Autodesk Fusion 360 part; units mm, degrees
(part 5 of 7)
  spline S7 degree 5 poles (-6.1927, -9.0912) (-6.1879, -9.089) (-6.1784, -9.0847) (-6.164, -9.0781) (-6.1449, -9.0692) (-6.1211, -9.0581) (-6.0974, -9.0469) (-6.0739, -9.0356) (-6.0504, -9.0242) (-6.0269, -9.0127) (-6.0036, -9.0011) (-5.9804, -8.9894) (-5.9573, -8.9776) (-5.9343, -8.9657) (-5.9113, -8.9538) (-5.8885, -8.9417) (-5.8657, -8.9295) (-5.8431, -8.9173) (-5.8206, -8.9049) (-5.7981, -8.8925) (-5.7758, -8.8799) (-5.7536, -8.8673) (-5.7314, -8.8545) (-5.7094, -8.8417) (-5.6875, -8.8288) (-5.6657, -8.8158) (-5.644, -8.8026) (-5.6224, -8.7894) (-5.6009, -8.7761) (-5.5795, -8.7627) (-5.5583, -8.7492) (-5.5371, -8.7356) (-5.5161, -8.7218) (-5.4952, -8.708) (-5.4744, -8.6941) (-5.4537, -8.6801) (-5.4331, -8.666) (-5.4127, -8.6518) (-5.3924, -8.6375) (-5.3722, -8.6231) (-5.3522, -8.6085) (-5.3323, -8.5939) (-5.3125, -8.5792) (-5.2928, -8.5643) (-5.2733, -8.5494) (-5.2539, -8.5343) (-5.2347, -8.5192) (-5.2156, -8.5039) (-5.1966, -8.4885) (-5.1778, -8.473) (-5.1592, -8.4574) (-5.1407, -8.4417) (-5.1224, -8.4258) (-5.1042, -8.4099) (-5.0862, -8.3938) (-5.0684, -8.3776) (-5.0507, -8.3612) (-5.0332, -8.3448) (-5.0159, -8.3283) (-4.9987, -8.3116) (-4.9818, -8.2947) (-4.9651, -8.2777) (-4.9487, -8.2605) (-4.9326, -8.2431) (-4.9167, -8.2256) (-4.901, -8.2079) (-4.8854, -8.1901) (-4.87, -8.1723) (-4.8548, -8.1543) (-4.84, -8.1361) (-4.8257, -8.1175) (-4.8149, -8.1023) (-4.8073, -8.0905) (-4.8024, -8.0825) (-4.8, -8.0785) knots -1 -1 -1 -1 -1 -1 -0.98571429 -0.97142857 -0.95714286 -0.94285714 -0.92857143 -0.91428571 -0.9 -0.88571429 -0.87142857 -0.85714286 -0.84285714 -0.82857143 -0.81428571 -0.8 -0.78571429 -0.77142857 -0.75714286 -0.74285714 -0.72857143 -0.71428571 -0.7 -0.68571429 -0.67142857 -0.65714286 -0.64285714 -0.62857143 -0.61428571 -0.6 -0.58571429 -0.57142857 -0.55714286 -0.54285714 -0.52857143 -0.51428571 -0.5 -0.48571429 -0.47142857 -0.45714286 -0.44285714 -0.42857143 -0.41428571 -0.4 -0.38571429 -0.37142857 -0.35714286 -0.34285714 -0.32857143 -0.31428571 -0.3 -0.28571429 -0.27142857 -0.25714286 -0.24285714 -0.22857143 -0.21428571 -0.2 -0.18571429 -0.17142857 -0.15714286 -0.14285714 -0.12857143 -0.11428571 -0.1 -0.08571429 -0.07142857 -0.05714286 -0.04285714 -0.02857143 -0.01428571 0 0 0 0 0 0
  line L7 (-4.8, -8.0785) -> (-4.6678, -7.856)
  arc A15 (-4.2652, -7.7464) -> (-4.6678, -7.856) centre (-4.4099, -8.0092) ccw
  arc A16 (-4.2652, -7.7464) -> (-3.76, -8.0038) centre (0, 0) ccw
  arc A17 (-3.6119, -8.3939) -> (-3.76, -8.0038) centre (-3.8875, -8.2754) ccw
  line L8 (-3.6119, -8.3939) -> (-3.7143, -8.6317)
  spline S8 degree 5 poles (-3.7143, -8.6317) (-3.7161, -8.636) (-3.7197, -8.6447) (-3.7247, -8.6577) (-3.7308, -8.6754) (-3.7374, -8.6979) (-3.7434, -8.7206) (-3.749, -8.7435) (-3.7544, -8.7664) (-3.7596, -8.7895) (-3.7647, -8.8126) (-3.7695, -8.8357) (-3.7741, -8.859) (-3.7784, -8.8824) (-3.7824, -8.9059) (-3.786, -8.9295) (-3.7894, -8.9532) (-3.7926, -8.9769) (-3.7956, -9.0007) (-3.7984, -9.0246) (-3.8011, -9.0486) (-3.8035, -9.0726) (-3.8058, -9.0967) (-3.8079, -9.1208) (-3.8097, -9.145) (-3.8114, -9.1693) (-3.8128, -9.1936) (-3.8141, -9.218) (-3.8153, -9.2424) (-3.8162, -9.2669) (-3.817, -9.2914) (-3.8176, -9.316) (-3.8181, -9.3406) (-3.8184, -9.3653) (-3.8185, -9.39) (-3.8185, -9.4147) (-3.8183, -9.4395) (-3.8179, -9.4644) (-3.8174, -9.4893) (-3.8168, -9.5142) (-3.8159, -9.5391) (-3.815, -9.5641) (-3.8139, -9.5892) (-3.8126, -9.6142) (-3.8112, -9.6394) (-3.8096, -9.6645) (-3.8079, -9.6897) (-3.806, -9.7149) (-3.804, -9.7401) (-3.8019, -9.7654) (-3.7996, -9.7907) (-3.7972, -9.816) (-3.7946, -9.8414) (-3.7919, -9.8668) (-3.7891, -9.8922) (-3.7861, -9.9176) (-3.783, -9.9431) (-3.7797, -9.9686) (-3.7763, -9.9941) (-3.7728, -10.0197) (-3.7692, -10.0452) (-3.7654, -10.0708) (-3.7614, -10.0964) (-3.7574, -10.1221) (-3.7532, -10.1477) (-3.7489, -10.1734) (-3.7444, -10.1991) (-3.7398, -10.2248) (-3.7351, -10.2506) (-3.7303, -10.2763) (-3.7253, -10.3021) (-3.7212, -10.3227) (-3.7181, -10.3382) (-3.716, -10.3485) (-3.7149, -10.3537) knots 0 0 0 0 0 0 0.01428571 0.02857143 0.04285714 0.05714286 0.07142857 0.08571429 0.1 0.11428571 0.12857143 0.14285714 0.15714286 0.17142857 0.18571429 0.2 0.21428571 0.22857143 0.24285714 0.25714286 0.27142857 0.28571429 0.3 0.31428571 0.32857143 0.34285714 0.35714286 0.37142857 0.38571429 0.4 0.41428571 0.42857143 0.44285714 0.45714286 0.47142857 0.48571429 0.5 0.51428571 0.52857143 0.54285714 0.55714286 0.57142857 0.58571429 0.6 0.61428571 0.62857143 0.64285714 0.65714286 0.67142857 0.68571429 0.7 0.71428571 0.72857143 0.74285714 0.75714286 0.77142857 0.78571429 0.8 0.81428571 0.82857143 0.84285714 0.85714286 0.87142857 0.88571429 0.9 0.91428571 0.92857143 0.94285714 0.95714286 0.97142857 0.98571429 1 1 1 1 1 1
  arc A18 (-3.7149, -10.3537) -> (-3.0803, -10.5599) centre (0, 0) ccw
  spline S9 degree 5 poles (-3.0803, -10.5599) (-3.0764, -10.5564) (-3.0687, -10.5492) (-3.057, -10.5385) (-3.0416, -10.5242) (-3.0224, -10.5063) (-3.0034, -10.4883) (-2.9844, -10.4703) (-2.9656, -10.4522) (-2.9469, -10.434) (-2.9283, -10.4158) (-2.9098, -10.3975) (-2.8915, -10.3791) (-2.8732, -10.3607) (-2.8551, -10.3422) (-2.8371, -10.3237) (-2.8193, -10.3051) (-2.8015, -10.2864) (-2.7839, -10.2677) (-2.7664, -10.249) (-2.7491, -10.2301) (-2.7318, -10.2112) (-2.7147, -10.1923) (-2.6977, -10.1733) (-2.6809, -10.1542) (-2.6642, -10.1351) (-2.6476, -10.1159) (-2.6311, -10.0966) (-2.6148, -10.0773) (-2.5986, -10.058) (-2.5826, -10.0386) (-2.5667, -10.0191) (-2.5509, -9.9995) (-2.5353, -9.9799) (-2.5198, -9.9603) (-2.5045, -9.9406) (-2.4893, -9.9208) (-2.4743, -9.901) (-2.4594, -9.8811) (-2.4446, -9.8611) (-2.43, -9.8411) (-2.4156, -9.821) (-2.4014, -9.8009) (-2.3873, -9.7807) (-2.3733, -9.7605) (-2.3595, -9.7402) (-2.3459, -9.7198) (-2.3325, -9.6994) (-2.3192, -9.6789) (-2.3061, -9.6584) (-2.2932, -9.6378) (-2.2805, -9.6171) (-2.2679, -9.5964) (-2.2556, -9.5755) (-2.2435, -9.5547) (-2.2315, -9.5338) (-2.2198, -9.5128) (-2.2082, -9.4917) (-2.1968, -9.4706) (-2.1856, -9.4495) (-2.1747, -9.4282) (-2.1641, -9.4069) (-2.1539, -9.3855) (-2.1439, -9.3639) (-2.1342, -9.3423) (-2.1248, -9.3207) (-2.1154, -9.299) (-2.1063, -9.2772) (-2.0974, -9.2554) (-2.0889, -9.2335) (-2.0811, -9.2115) (-2.0755, -9.1936) (-2.0719, -9.1801) (-2.0697, -9.171) (-2.0687, -9.1664) knots -1 -1 -1 -1 -1 -1 -0.98571429 -0.97142857 -0.95714286 -0.94285714 -0.92857143 -0.91428571 -0.9 -0.88571429 -0.87142857 -0.85714286 -0.84285714 -0.82857143 -0.81428571 -0.8 -0.78571429 -0.77142857 -0.75714286 -0.74285714 -0.72857143 -0.71428571 -0.7 -0.68571429 -0.67142857 -0.65714286 -0.64285714 -0.62857143 -0.61428571 -0.6 -0.58571429 -0.57142857 -0.55714286 -0.54285714 -0.52857143 -0.51428571 -0.5 -0.48571429 -0.47142857 -0.45714286 -0.44285714 -0.42857143 -0.41428571 -0.4 -0.38571429 -0.37142857 -0.35714286 -0.34285714 -0.32857143 -0.31428571 -0.3 -0.28571429 -0.27142857 -0.25714286 -0.24285714 -0.22857143 -0.21428571 -0.2 -0.18571429 -0.17142857 -0.15714286 -0.14285714 -0.12857143 -0.11428571 -0.1 -0.08571429 -0.07142857 -0.05714286 -0.04285714 -0.02857143 -0.01428571 0 0 0 0 0 0
  line L9 (-2.0687, -9.1664) -> (-2.0117, -8.9139)
  arc A19 (-1.6627, -8.6853) -> (-2.0117, -8.9139) centre (-1.7191, -8.9799) ccw
  arc A20 (-1.6627, -8.6853) -> (-1.1026, -8.774) centre (0, 0) ccw
  arc A21 (-0.8413, -9.0993) -> (-1.1026, -8.774) centre (-1.14, -9.0716) ccw
  line L10 (-0.8413, -9.0993) -> (-0.8651, -9.357)
  spline S10 degree 5 poles (-0.8651, -9.357) (-0.8655, -9.3617) (-0.8663, -9.371) (-0.867, -9.385) (-0.8673, -9.4037) (-0.8667, -9.4271) (-0.8654, -9.4506) (-0.8636, -9.474) (-0.8616, -9.4975) (-0.8595, -9.5211) (-0.8572, -9.5446) (-0.8546, -9.5681) (-0.8518, -9.5917) (-0.8487, -9.6152) (-0.8452, -9.6388) (-0.8414, -9.6624) (-0.8373, -9.686) (-0.833, -9.7095) (-0.8285, -9.7331) (-0.8238, -9.7567) (-0.8189, -9.7803) (-0.8138, -9.8039) (-0.8085, -9.8275) (-0.803, -9.8511) (-0.7973, -9.8747) (-0.7914, -9.8983) (-0.7853, -9.9219) (-0.779, -9.9454) (-0.7725, -9.969) (-0.7658, -9.9926) (-0.759, -10.0162) (-0.752, -10.0397) (-0.7448, -10.0633) (-0.7375, -10.0868) (-0.73, -10.1104) (-0.7223, -10.1339) (-0.7144, -10.1574) (-0.7064, -10.181) (-0.6982, -10.2045) (-0.6899, -10.228) (-0.6814, -10.2515) (-0.6728, -10.2749) (-0.664, -10.2984) (-0.655, -10.3218) (-0.6459, -10.3453) (-0.6367, -10.3687) (-0.6273, -10.3921) (-0.6177, -10.4155) (-0.608, -10.4389) (-0.5982, -10.4623) (-0.5882, -10.4857) (-0.578, -10.509) (-0.5678, -10.5323) (-0.5573, -10.5556) (-0.5468, -10.5789) (-0.5361, -10.6022) (-0.5252, -10.6255) (-0.5143, -10.6487) (-0.5032, -10.6719) (-0.4919, -10.6951) (-0.4805, -10.7183) (-0.469, -10.7415) (-0.4574, -10.7646) (-0.4456, -10.7878) (-0.4337, -10.8109) (-0.4216, -10.834) (-0.4094, -10.857) (-0.3971, -10.8801) (-0.3847, -10.9031) (-0.3721, -10.9261) (-0.3594, -10.9491) (-0.3492, -10.9674) (-0.3414, -10.9812) (-0.3362, -10.9904) (-0.3336, -10.9949) knots 0 0 0 0 0 0 0.01428571 0.02857143 0.04285714 0.05714286 0.07142857 0.08571429 0.1 0.11428571 0.12857143 0.14285714 0.15714286 0.17142857 0.18571429 0.2 0.21428571 0.22857143 0.24285714 0.25714286 0.27142857 0.28571429 0.3 0.31428571 0.32857143 0.34285714 0.35714286 0.37142857 0.38571429 0.4 0.41428571 0.42857143 0.44285714 0.45714286 0.47142857 0.48571429 0.5 0.51428571 0.52857143 0.54285714 0.55714286 0.57142857 0.58571429 0.6 0.61428571 0.62857143 0.64285714 0.65714286 0.67142857 0.68571429 0.7 0.71428571 0.72857143 0.74285714 0.75714286 0.77142857 0.78571429 0.8 0.81428571 0.82857143 0.84285714 0.85714286 0.87142857 0.88571429 0.9 0.91428571 0.92857143 0.94285714 0.95714286 0.97142857 0.98571429 1 1 1 1 1 1
  arc A22 (-0.3336, -10.9949) -> (0.3336, -10.9949) centre (0, 0) ccw
  spline S11 degree 5 poles (0.3336, -10.9949) (0.3362, -10.9904) (0.3414, -10.9812) (0.3492, -10.9674) (0.3594, -10.9491) (0.3721, -10.9261) (0.3847, -10.9031) (0.3971, -10.8801) (0.4094, -10.857) (0.4216, -10.834) (0.4337, -10.8109) (0.4456, -10.7878) (0.4574, -10.7646) (0.469, -10.7415) (0.4805, -10.7183) (0.4919, -10.6951) (0.5032, -10.6719) (0.5143, -10.6487) (0.5252, -10.6255) (0.5361, -10.6022) (0.5468, -10.5789) (0.5573, -10.5556) (0.5678, -10.5323) (0.578, -10.509) (0.5882, -10.4857) (0.5982, -10.4623) (0.608, -10.4389) (0.6177, -10.4155) (0.6273, -10.3921) (0.6367, -10.3687) (0.6459, -10.3453) (0.655, -10.3218) (0.664, -10.2984) (0.6728, -10.2749) (0.6814, -10.2515) (0.6899, -10.228) (0.6982, -10.2045) (0.7064, -10.181) (0.7144, -10.1574) (0.7223, -10.1339) (0.73, -10.1104) (0.7375, -10.0868) (0.7448, -10.0633) (0.752, -10.0397) (0.759, -10.0162) (0.7658, -9.9926) (0.7725, -9.969) (0.779, -9.9454) (0.7853, -9.9219) (0.7914, -9.8983) (0.7973, -9.8747) (0.803, -9.8511) (0.8085, -9.8275) (0.8138, -9.8039) (0.8189, -9.7803) (0.8238, -9.7567) (0.8285, -9.7331) (0.833, -9.7095) (0.8373, -9.686) (0.8414, -9.6624) (0.8452, -9.6388) (0.8487, -9.6152) (0.8518, -9.5917) (0.8546, -9.5681) (0.8572, -9.5446) (0.8595, -9.5211) (0.8616, -9.4975) (0.8636, -9.474) (0.8654, -9.4506) (0.8667, -9.4271) (0.8673, -9.4037) (0.867, -9.385) (0.8663, -9.371) (0.8655, -9.3617) (0.8651, -9.357) knots -1 -1 -1 -1 -1 -1 -0.98571429 -0.97142857 -0.95714286 -0.94285714 -0.92857143 -0.91428571 -0.9 -0.88571429 -0.87142857 -0.85714286 -0.84285714 -0.82857143 -0.81428571 -0.8 -0.78571429 -0.77142857 -0.75714286 -0.74285714 -0.72857143 -0.71428571 -0.7 -0.68571429 -0.67142857 -0.65714286 -0.64285714 -0.62857143 -0.61428571 -0.6 -0.58571429 -0.57142857 -0.55714286 -0.54285714 -0.52857143 -0.51428571 -0.5 -0.48571429 -0.47142857 -0.45714286 -0.44285714 -0.42857143 -0.41428571 -0.4 -0.38571429 -0.37142857 -0.35714286 -0.34285714 -0.32857143 -0.31428571 -0.3 -0.28571429 -0.27142857 -0.25714286 -0.24285714 -0.22857143 -0.21428571 -0.2 -0.18571429 -0.17142857 -0.15714286 -0.14285714 -0.12857143 -0.11428571 -0.1 -0.08571429 -0.07142857 -0.05714286 -0.04285714 -0.02857143 -0.01428571 0 0 0 0 0 0
  line L11 (0.8651, -9.357) -> (0.8413, -9.0993)
  arc A23 (1.1026, -8.774) -> (0.8413, -9.0993) centre (1.14, -9.0716) ccw
  arc A24 (1.1026, -8.774) -> (1.6627, -8.6853) centre (0, 0) ccw
  arc A25 (2.0117, -8.9139) -> (1.6627, -8.6853) centre (1.7191, -8.9799) ccw
  line L12 (2.0117, -8.9139) -> (2.0687, -9.1664)
  spline S12 degree 5 poles (2.0687, -9.1664) (2.0697, -9.171) (2.0719, -9.1801) (2.0755, -9.1936) (2.0811, -9.2115) (2.0889, -9.2335) (2.0974, -9.2554) (2.1063, -9.2772) (2.1154, -9.299) (2.1248, -9.3207) (2.1342, -9.3423) (2.1439, -9.3639) (2.1539, -9.3855) (2.1641, -9.4069) (2.1747, -9.4282) (2.1856, -9.4495) (2.1968, -9.4706) (2.2082, -9.4917) (2.2198, -9.5128) (2.2315, -9.5338) (2.2435, -9.5547) (2.2556, -9.5755) (2.2679, -9.5964) (2.2805, -9.6171) (2.2932, -9.6378) (2.3061, -9.6584) (2.3192, -9.6789) (2.3325, -9.6994) (2.3459, -9.7198) (2.3595, -9.7402) (2.3733, -9.7605) (2.3873, -9.7807) (2.4014, -9.8009) (2.4156, -9.821) (2.43, -9.8411) (2.4446, -9.8611) (2.4594, -9.8811) (2.4743, -9.901) (2.4893, -9.9208) (2.5045, -9.9406) (2.5198, -9.9603) (2.5353, -9.9799) (2.5509, -9.9995) (2.5667, -10.0191) (2.5826, -10.0386) (2.5986, -10.058) (2.6148, -10.0773) (2.6311, -10.0966) (2.6476, -10.1159) (2.6642, -10.1351) (2.6809, -10.1542) (2.6977, -10.1733) (2.7147, -10.1923) (2.7318, -10.2112) (2.7491, -10.2301) (2.7664, -10.249) (2.7839, -10.2677) (2.8015, -10.2864) (2.8193, -10.3051) (2.8371, -10.3237) (2.8551, -10.3422) (2.8732, -10.3607) (2.8915, -10.3791) (2.9098, -10.3975) (2.9283, -10.4158) (2.9469, -10.434) (2.9656, -10.4522) (2.9844, -10.4703) (3.0034, -10.4883) (3.0224, -10.5063) (3.0416, -10.5242) (3.057, -10.5385) (3.0687, -10.5492) (3.0764, -10.5564) (3.0803, -10.5599) knots 0 0 0 0 0 0 0.01428571 0.02857143 0.04285714 0.05714286 0.07142857 0.08571429 0.1 0.11428571 0.12857143 0.14285714 0.15714286 0.17142857 0.18571429 0.2 0.21428571 0.22857143 0.24285714 0.25714286 0.27142857 0.28571429 0.3 0.31428571 0.32857143 0.34285714 0.35714286 0.37142857 0.38571429 0.4 0.41428571 0.42857143 0.44285714 0.45714286 0.47142857 0.48571429 0.5 0.51428571 0.52857143 0.54285714 0.55714286 0.57142857 0.58571429 0.6 0.61428571 0.62857143 0.64285714 0.65714286 0.67142857 0.68571429 0.7 0.71428571 0.72857143 0.74285714 0.75714286 0.77142857 0.78571429 0.8 0.81428571 0.82857143 0.84285714 0.85714286 0.87142857 0.88571429 0.9 0.91428571 0.92857143 0.94285714 0.95714286 0.97142857 0.98571429 1 1 1 1 1 1
  arc A26 (3.0803, -10.5599) -> (3.7149, -10.3537) centre (0, 0) ccw
  spline S13 degree 5 poles (3.7149, -10.3537) (3.716, -10.3485) (3.7181, -10.3382) (3.7212, -10.3227) (3.7253, -10.3021) (3.7303, -10.2763) (3.7351, -10.2506) (3.7398, -10.2248) (3.7444, -10.1991) (3.7489, -10.1734) (3.7532, -10.1477) (3.7574, -10.1221) (3.7614, -10.0964) (3.7654, -10.0708) (3.7692, -10.0452) (3.7728, -10.0197) (3.7763, -9.9941) (3.7797, -9.9686) (3.783, -9.9431) (3.7861, -9.9176) (3.7891, -9.8922) (3.7919, -9.8668) (3.7946, -9.8414) (3.7972, -9.816) (3.7996, -9.7907) (3.8019, -9.7654) (3.804, -9.7401) (3.806, -9.7149) (3.8079, -9.6897) (3.8096, -9.6645) (3.8112, -9.6394) (3.8126, -9.6142) (3.8139, -9.5892) (3.815, -9.5641) (3.8159, -9.5391) (3.8168, -9.5142) (3.8174, -9.4893) (3.8179, -9.4644) (3.8183, -9.4395) (3.8185, -9.4147) (3.8185, -9.39) (3.8184, -9.3653) (3.8181, -9.3406) (3.8176, -9.316) (3.817, -9.2914) (3.8162, -9.2669) (3.8153, -9.2424) (3.8141, -9.218) (3.8128, -9.1936) (3.8114, -9.1693) (3.8097, -9.145) (3.8079, -9.1208) (3.8058, -9.0967) (3.8035, -9.0726) (3.8011, -9.0486) (3.7984, -9.0246) (3.7956, -9.0007) (3.7926, -8.9769) (3.7894, -8.9532) (3.786, -8.9295) (3.7824, -8.9059) (3.7784, -8.8824) (3.7741, -8.859) (3.7695, -8.8357) (3.7647, -8.8126) (3.7596, -8.7895) (3.7544, -8.7664) (3.749, -8.7435) (3.7434, -8.7206) (3.7374, -8.6979) (3.7308, -8.6754) (3.7247, -8.6577) (3.7197, -8.6447) (3.7161, -8.636) (3.7143, -8.6317) knots -1 -1 -1 -1 -1 -1 -0.98571429 -0.97142857 -0.95714286 -0.94285714 -0.92857143 -0.91428571 -0.9 -0.88571429 -0.87142857 -0.85714286 -0.84285714 -0.82857143 -0.81428571 -0.8 -0.78571429 -0.77142857 -0.75714286 -0.74285714 -0.72857143 -0.71428571 -0.7 -0.68571429 -0.67142857 -0.65714286 -0.64285714 -0.62857143 -0.61428571 -0.6 -0.58571429 -0.57142857 -0.55714286 -0.54285714 -0.52857143 -0.51428571 -0.5 -0.48571429 -0.47142857 -0.45714286 -0.44285714 -0.42857143 -0.41428571 -0.4 -0.38571429 -0.37142857 -0.35714286 -0.34285714 -0.32857143 -0.31428571 -0.3 -0.28571429 -0.27142857 -0.25714286 -0.24285714 -0.22857143 -0.21428571 -0.2 -0.18571429 -0.17142857 -0.15714286 -0.14285714 -0.12857143 -0.11428571 -0.1 -0.08571429 -0.07142857 -0.05714286 -0.04285714 -0.02857143 -0.01428571 0 0 0 0 0 0
  line L13 (3.7143, -8.6317) -> (3.6119, -8.3939)
  arc A27 (3.76, -8.0038) -> (3.6119, -8.3939) centre (3.8875, -8.2754) ccw
  arc A28 (3.76, -8.0038) -> (4.2652, -7.7464) centre (0, 0) ccw
  arc A29 (4.6678, -7.856) -> (4.2652, -7.7464) centre (4.4099, -8.0092) ccw
  line L14 (4.6678, -7.856) -> (4.8, -8.0785)
  spline S14 degree 5 poles (4.8, -8.0785) (4.8024, -8.0825) (4.8073, -8.0905) (4.8149, -8.1023) (4.8257, -8.1175) (4.84, -8.1361) (4.8548, -8.1543) (4.87, -8.1723) (4.8854, -8.1901) (4.901, -8.2079) (4.9167, -8.2256) (4.9326, -8.2431) (4.9487, -8.2605) (4.9651, -8.2777) (4.9818, -8.2947) (4.9987, -8.3116) (5.0159, -8.3283) (5.0332, -8.3448) (5.0507, -8.3612) (5.0684, -8.3776) (5.0862, -8.3938) (5.1042, -8.4099) (5.1224, -8.4258) (5.1407, -8.4417) (5.1592, -8.4574) (5.1778, -8.473) (5.1966, -8.4885) (5.2156, -8.5039) (5.2347, -8.5192) (5.2539, -8.5343) (5.2733, -8.5494) (5.2928, -8.5643) (5.3125, -8.5792) (5.3323, -8.5939) (5.3522, -8.6085) (5.3722, -8.6231) (5.3924, -8.6375) (5.4127, -8.6518) (5.4331, -8.666) (5.4537, -8.6801) (5.4744, -8.6941) (5.4952, -8.708) (5.5161, -8.7218) (5.5371, -8.7356) (5.5583, -8.7492) (5.5795, -8.7627) (5.6009, -8.7761) (5.6224, -8.7894) (5.644, -8.8026) (5.6657, -8.8158) (5.6875, -8.8288) (5.7094, -8.8417) (5.7314, -8.8545) (5.7536, -8.8673) (5.7758, -8.8799) (5.7981, -8.8925) (5.8206, -8.9049) (5.8431, -8.9173) (5.8657, -8.9295) (5.8885, -8.9417) (5.9113, -8.9538) (5.9343, -8.9657) (5.9573, -8.9776) (5.9804, -8.9894) (6.0036, -9.0011) (6.0269, -9.0127) (6.0504, -9.0242) (6.0739, -9.0356) (6.0974, -9.0469) (6.1211, -9.0581) (6.1449, -9.0692) (6.164, -9.0781) (6.1784, -9.0847) (6.1879, -9.089) (6.1927, -9.0912) knots 0 0 0 0 0 0 0.01428571 0.02857143 0.04285714 0.05714286 0.07142857 0.08571429 0.1 0.11428571 0.12857143 0.14285714 0.15714286 0.17142857 0.18571429 0.2 0.21428571 0.22857143 0.24285714 0.25714286 0.27142857 0.28571429 0.3 0.31428571 0.32857143 0.34285714 0.35714286 0.37142857 0.38571429 0.4 0.41428571 0.42857143 0.44285714 0.45714286 0.47142857 0.48571429 0.5 0.51428571 0.52857143 0.54285714 0.55714286 0.57142857 0.58571429 0.6 0.61428571 0.62857143 0.64285714 0.65714286 0.67142857 0.68571429 0.7 0.71428571 0.72857143 0.74285714 0.75714286 0.77142857 0.78571429 0.8 0.81428571 0.82857143 0.84285714 0.85714286 0.87142857 0.88571429 0.9 0.91428571 0.92857143 0.94285714 0.95714286 0.97142857 0.98571429 1 1 1 1 1 1
  arc A30 (6.1927, -9.0912) -> (6.7326, -8.699) centre (0, 0) ccw
  spline S15 degree 5 poles (6.7326, -8.699) (6.732, -8.6937) (6.7308, -8.6833) (6.729, -8.6676) (6.7265, -8.6467) (6.7233, -8.6207) (6.7199, -8.5947) (6.7164, -8.5687) (6.7128, -8.5429) (6.7091, -8.517) (6.7053, -8.4913) (6.7014, -8.4656) (6.6973, -8.4399) (6.6931, -8.4144) (6.6888, -8.3889) (6.6844, -8.3634) (6.6799, -8.338) (6.6752, -8.3127) (6.6704, -8.2875) (6.6655, -8.2623) (6.6605, -8.2371) (6.6553, -8.2121) (6.6501, -8.1871) (6.6447, -8.1622) (6.6391, -8.1374) (6.6335, -8.1126) (6.6277, -8.0879) (6.6218, -8.0633) (6.6158, -8.0387) (6.6096, -8.0143) (6.6034, -7.9899) (6.5969, -7.9655) (6.5904, -7.9413) (6.5837, -7.9171) (6.5769, -7.8931) (6.57, -7.8691) (6.5629, -7.8452) (6.5557, -7.8213) (6.5484, -7.7976) (6.5409, -7.774) (6.5333, -7.7504) (6.5255, -7.7269) (6.5176, -7.7036) (6.5096, -7.6803) (6.5014, -7.6571) (6.4931, -7.634) (6.4846, -7.6111) (6.476, -7.5882) (6.4672, -7.5654) (6.4583, -7.5427) (6.4492, -7.5202) (6.44, -7.4977) (6.4306, -7.4754) (6.421, -7.4532) (6.4112, -7.4311) (6.4013, -7.4092) (6.3912, -7.3873) (6.381, -7.3656) (6.3706, -7.344) (6.3601, -7.3225) (6.3493, -7.3012) (6.3383, -7.28) (6.327, -7.2591) (6.3154, -7.2384) (6.3036, -7.2179) (6.2917, -7.1975) (6.2796, -7.1772) (6.2674, -7.157) (6.255, -7.137) (6.2423, -7.1173) (6.229, -7.098) (6.2178, -7.083) (6.209, -7.0721) (6.2029, -7.065) (6.1998, -7.0615) knots -1 -1 -1 -1 -1 -1 -0.98571429 -0.97142857 -0.95714286 -0.94285714 -0.92857143 -0.91428571 -0.9 -0.88571429 -0.87142857 -0.85714286 -0.84285714 -0.82857143 -0.81428571 -0.8 -0.78571429 -0.77142857 -0.75714286 -0.74285714 -0.72857143 -0.71428571 -0.7 -0.68571429 -0.67142857 -0.65714286 -0.64285714 -0.62857143 -0.61428571 -0.6 -0.58571429 -0.57142857 -0.55714286 -0.54285714 -0.52857143 -0.51428571 -0.5 -0.48571429 -0.47142857 -0.45714286 -0.44285714 -0.42857143 -0.41428571 -0.4 -0.38571429 -0.37142857 -0.35714286 -0.34285714 -0.32857143 -0.31428571 -0.3 -0.28571429 -0.27142857 -0.25714286 -0.24285714 -0.22857143 -0.21428571 -0.2 -0.18571429 -0.17142857 -0.15714286 -0.14285714 -0.12857143 -0.11428571 -0.1 -0.08571429 -0.07142857 -0.05714286 -0.04285714 -0.02857143 -0.01428571 0 0 0 0 0 0
  line L15 (6.1998, -7.0615) -> (6.029, -6.867)
  arc A31 (6.0492, -6.4502) -> (6.029, -6.867) centre (6.2545, -6.669) ccw
  arc A32 (6.0492, -6.4502) -> (6.4502, -6.0492) centre (0, 0) ccw
  arc A33 (6.867, -6.029) -> (6.4502, -6.0492) centre (6.669, -6.2545) ccw
  line L16 (6.867, -6.029) -> (7.0615, -6.1998)
  spline S16 degree 5 poles (7.0615, -6.1998) (7.065, -6.2029) (7.0721, -6.209) (7.083, -6.2178) (7.098, -6.229) (7.1173, -6.2423) (7.137, -6.255) (7.157, -6.2674) (7.1772, -6.2796) (7.1975, -6.2917) (7.2179, -6.3036) (7.2384, -6.3154) (7.2591, -6.327) (7.28, -6.3383) (7.3012, -6.3493) (7.3225, -6.3601) (7.344, -6.3706) (7.3656, -6.381) (7.3873, -6.3912) (7.4092, -6.4013) (7.4311, -6.4112) (7.4532, -6.421) (7.4754, -6.4306) (7.4977, -6.44) (7.5202, -6.4492) (7.5427, -6.4583) (7.5654, -6.4672) (7.5882, -6.476) (7.6111, -6.4846) (7.634, -6.4931) (7.6571, -6.5014) (7.6803, -6.5096) (7.7036, -6.5176) (7.7269, -6.5255) (7.7504, -6.5333) (7.774, -6.5409) (7.7976, -6.5484) (7.8213, -6.5557) (7.8452, -6.5629) (7.8691, -6.57) (7.8931, -6.5769) (7.9171, -6.5837) (7.9413, -6.5904) (7.9655, -6.5969) (7.9899, -6.6034) (8.0143, -6.6096) (8.0387, -6.6158) (8.0633, -6.6218) (8.0879, -6.6277) (8.1126, -6.6335) (8.1374, -6.6391) (8.1622, -6.6447) (8.1871, -6.6501) (8.2121, -6.6553) (8.2371, -6.6605) (8.2623, -6.6655) (8.2875, -6.6704) (8.3127, -6.6752) (8.338, -6.6799) (8.3634, -6.6844) (8.3889, -6.6888) (8.4144, -6.6931) (8.4399, -6.6973) (8.4656, -6.7014) (8.4913, -6.7053) (8.517, -6.7091) (8.5429, -6.7128) (8.5687, -6.7164) (8.5947, -6.7199) (8.6207, -6.7233) (8.6467, -6.7265) (8.6676, -6.729) (8.6833, -6.7308) (8.6937, -6.732) (8.699, -6.7326) knots 0 0 0 0 0 0 0.01428571 0.02857143 0.04285714 0.05714286 0.07142857 0.08571429 0.1 0.11428571 0.12857143 0.14285714 0.15714286 0.17142857 0.18571429 0.2 0.21428571 0.22857143 0.24285714 0.25714286 0.27142857 0.28571429 0.3 0.31428571 0.32857143 0.34285714 0.35714286 0.37142857 0.38571429 0.4 0.41428571 0.42857143 0.44285714 0.45714286 0.47142857 0.48571429 0.5 0.51428571 0.52857143 0.54285714 0.55714286 0.57142857 0.58571429 0.6 0.61428571 0.62857143 0.64285714 0.65714286 0.67142857 0.68571429 0.7 0.71428571 0.72857143 0.74285714 0.75714286 0.77142857 0.78571429 0.8 0.81428571 0.82857143 0.84285714 0.85714286 0.87142857 0.88571429 0.9 0.91428571 0.92857143 0.94285714 0.95714286 0.97142857 0.98571429 1 1 1 1 1 1
  arc A34 (8.699, -6.7326) -> (9.0912, -6.1927) centre (0, 0) ccw
  spline S17 degree 5 poles (9.0912, -6.1927) (9.089, -6.1879) (9.0847, -6.1784) (9.0781, -6.164) (9.0692, -6.1449) (9.0581, -6.1211) (9.0469, -6.0974) (9.0356, -6.0739) (9.0242, -6.0504) (9.0127, -6.0269) (9.0011, -6.0036) (8.9894, -5.9804) (8.9776, -5.9573) (8.9657, -5.9343) (8.9538, -5.9113) (8.9417, -5.8885) (8.9295, -5.8657) (8.9173, -5.8431) (8.9049, -5.8206) (8.8925, -5.7981) (8.8799, -5.7758) (8.8673, -5.7536) (8.8545, -5.7314) (8.8417, -5.7094) (8.8288, -5.6875) (8.8158, -5.6657) (8.8026, -5.644) (8.7894, -5.6224) (8.7761, -5.6009) (8.7627, -5.5795) (8.7492, -5.5583) (8.7356, -5.5371) (8.7218, -5.5161) (8.708, -5.4952) (8.6941, -5.4744) (8.6801, -5.4537) (8.666, -5.4331) (8.6518, -5.4127) (8.6375, -5.3924) (8.6231, -5.3722) (8.6085, -5.3522) (8.5939, -5.3323) (8.5792, -5.3125) (8.5643, -5.2928) (8.5494, -5.2733) (8.5343, -5.2539) (8.5192, -5.2347) (8.5039, -5.2156) (8.4885, -5.1966) (8.473, -5.1778) (8.4574, -5.1592) (8.4417, -5.1407) (8.4258, -5.1224) (8.4099, -5.1042) (8.3938, -5.0862) (8.3776, -5.0684) (8.3612, -5.0507) (8.3448, -5.0332) (8.3283, -5.0159) (8.3116, -4.9987) (8.2947, -4.9818) (8.2777, -4.9651) (8.2605, -4.9487) (8.2431, -4.9326) (8.2256, -4.9167) (8.2079, -4.901) (8.1901, -4.8854) (8.1723, -4.87) (8.1543, -4.8548) (8.1361, -4.84) (8.1175, -4.8257) (8.1023, -4.8149) (8.0905, -4.8073) (8.0825, -4.8024) (8.0785, -4.8) knots -1 -1 -1 -1 -1 -1 -0.98571429 -0.97142857 -0.95714286 -0.94285714 -0.92857143 -0.91428571 -0.9 -0.88571429 -0.87142857 -0.85714286 -0.84285714 -0.82857143 -0.81428571 -0.8 -0.78571429 -0.77142857 -0.75714286 -0.74285714 -0.72857143 -0.71428571 -0.7 -0.68571429 -0.67142857 -0.65714286 -0.64285714 -0.62857143 -0.61428571 -0.6 -0.58571429 -0.57142857 -0.55714286 -0.54285714 -0.52857143 -0.51428571 -0.5 -0.48571429 -0.47142857 -0.45714286 -0.44285714 -0.42857143 -0.41428571 -0.4 -0.38571429 -0.37142857 -0.35714286 -0.34285714 -0.32857143 -0.31428571 -0.3 -0.28571429 -0.27142857 -0.25714286 -0.24285714 -0.22857143 -0.21428571 -0.2 -0.18571429 -0.17142857 -0.15714286 -0.14285714 -0.12857143 -0.11428571 -0.1 -0.08571429 -0.07142857 -0.05714286 -0.04285714 -0.02857143 -0.01428571 0 0 0 0 0 0
  line L17 (8.0785, -4.8) -> (7.856, -4.6678)
  arc A35 (7.7464, -4.2652) -> (7.856, -4.6678) centre (8.0092, -4.4099) ccw
  arc A36 (7.7464, -4.2652) -> (8.0038, -3.76) centre (0, 0) ccw
  arc A37 (8.3939, -3.6119) -> (8.0038, -3.76) centre (8.2754, -3.8875) ccw
  line L18 (8.3939, -3.6119) -> (8.6317, -3.7143)
  spline S18 degree 5 poles (8.6317, -3.7143) (8.636, -3.7161) (8.6447, -3.7197) (8.6577, -3.7247) (8.6754, -3.7308) (8.6979, -3.7374) (8.7206, -3.7434) (8.7435, -3.749) (8.7664, -3.7544) (8.7895, -3.7596) (8.8126, -3.7647) (8.8357, -3.7695) (8.859, -3.7741) (8.8824, -3.7784) (8.9059, -3.7824) (8.9295, -3.786) (8.9532, -3.7894) (8.9769, -3.7926) (9.0007, -3.7956) (9.0246, -3.7984) (9.0486, -3.8011) (9.0726, -3.8035) (9.0967, -3.8058) (9.1208, -3.8079) (9.145, -3.8097) (9.1693, -3.8114) (9.1936, -3.8128) (9.218, -3.8141) (9.2424, -3.8153) (9.2669, -3.8162) (9.2914, -3.817) (9.316, -3.8176) (9.3406, -3.8181) (9.3653, -3.8184) (9.39, -3.8185) (9.4147, -3.8185) (9.4395, -3.8183) (9.4644, -3.8179) (9.4893, -3.8174) (9.5142, -3.8168) (9.5391, -3.8159) (9.5641, -3.815) (9.5892, -3.8139) (9.6142, -3.8126) (9.6394, -3.8112) (9.6645, -3.8096) (9.6897, -3.8079) (9.7149, -3.806) (9.7401, -3.804) (9.7654, -3.8019) (9.7907, -3.7996) (9.816, -3.7972) (9.8414, -3.7946) (9.8668, -3.7919) (9.8922, -3.7891) (9.9176, -3.7861) (9.9431, -3.783) (9.9686, -3.7797) (9.9941, -3.7763) (10.0197, -3.7728) (10.0452, -3.7692) (10.0708, -3.7654) (10.0964, -3.7614) (10.1221, -3.7574) (10.1477, -3.7532) (10.1734, -3.7489) (10.1991, -3.7444) (10.2248, -3.7398) (10.2506, -3.7351) (10.2763, -3.7303) (10.3021, -3.7253) (10.3227, -3.7212) (10.3382, -3.7181) (10.3485, -3.716) (10.3537, -3.7149) knots 0 0 0 0 0 0 0.01428571 0.02857143 0.04285714 0.05714286 0.07142857 0.08571429 0.1 0.11428571 0.12857143 0.14285714 0.15714286 0.17142857 0.18571429 0.2 0.21428571 0.22857143 0.24285714 0.25714286 0.27142857 0.28571429 0.3 0.31428571 0.32857143 0.34285714 0.35714286 0.37142857 0.38571429 0.4 0.41428571 0.42857143 0.44285714 0.45714286 0.47142857 0.48571429 0.5 0.51428571 0.52857143 0.54285714 0.55714286 0.57142857 0.58571429 0.6 0.61428571 0.62857143 0.64285714 0.65714286 0.67142857 0.68571429 0.7 0.71428571 0.72857143 0.74285714 0.75714286 0.77142857 0.78571429 0.8 0.81428571 0.82857143 0.84285714 0.85714286 0.87142857 0.88571429 0.9 0.91428571 0.92857143 0.94285714 0.95714286 0.97142857 0.98571429 1 1 1 1 1 1
  arc A38 (10.3537, -3.7149) -> (10.5599, -3.0803) centre (0, 0) ccw
  spline S19 degree 5 poles (10.5599, -3.0803) (10.5564, -3.0764) (10.5492, -3.0687) (10.5385, -3.057) (10.5242, -3.0416) (10.5063, -3.0224) (10.4883, -3.0034) (10.4703, -2.9844) (10.4522, -2.9656) (10.434, -2.9469) (10.4158, -2.9283) (10.3975, -2.9098) (10.3791, -2.8915) (10.3607, -2.8732) (10.3422, -2.8551) (10.3237, -2.8371) (10.3051, -2.8193) (10.2864, -2.8015) (10.2677, -2.7839) (10.249, -2.7664) (10.2301, -2.7491) (10.2112, -2.7318) (10.1923, -2.7147) (10.1733, -2.6977) (10.1542, -2.6809) (10.1351, -2.6642) (10.1159, -2.6476) (10.0966, -2.6311) (10.0773, -2.6148) (10.058, -2.5986) (10.0386, -2.5826) (10.0191, -2.5667) (9.9995, -2.5509) (9.9799, -2.5353) (9.9603, -2.5198) (9.9406, -2.5045) (9.9208, -2.4893) (9.901, -2.4743) (9.8811, -2.4594) (9.8611, -2.4446) (9.8411, -2.43) (9.821, -2.4156) (9.8009, -2.4014) (9.7807, -2.3873) (9.7605, -2.3733) (9.7402, -2.3595) (9.7198, -2.3459) (9.6994, -2.3325) (9.6789, -2.3192) (9.6584, -2.3061) (9.6378, -2.2932) (9.6171, -2.2805) (9.5964, -2.2679) (9.5755, -2.2556) (9.5547, -2.2435) (9.5338, -2.2315) (9.5128, -2.2198) (9.4917, -2.2082) (9.4706, -2.1968) (9.4495, -2.1856) (9.4282, -2.1747) (9.4069, -2.1641) (9.3855, -2.1539) (9.3639, -2.1439) (9.3423, -2.1342) (9.3207, -2.1248) (9.299, -2.1154) (9.2772, -2.1063) (9.2554, -2.0974) (9.2335, -2.0889) (9.2115, -2.0811) (9.1936, -2.0755) (9.1801, -2.0719) (9.171, -2.0697) (9.1664, -2.0687) knots -1 -1 -1 -1 -1 -1 -0.98571429 -0.97142857 -0.95714286 -0.94285714 -0.92857143 -0.91428571 -0.9 -0.88571429 -0.87142857 -0.85714286 -0.84285714 -0.82857143 -0.81428571 -0.8 -0.78571429 -0.77142857 -0.75714286 -0.74285714 -0.72857143 -0.71428571 -0.7 -0.68571429 -0.67142857 -0.65714286 -0.64285714 -0.62857143 -0.61428571 -0.6 -0.58571429 -0.57142857 -0.55714286 -0.54285714 -0.52857143 -0.51428571 -0.5 -0.48571429 -0.47142857 -0.45714286 -0.44285714 -0.42857143 -0.41428571 -0.4 -0.38571429 -0.37142857 -0.35714286 -0.34285714 -0.32857143 -0.31428571 -0.3 -0.28571429 -0.27142857 -0.25714286 -0.24285714 -0.22857143 -0.21428571 -0.2 -0.18571429 -0.17142857 -0.15714286 -0.14285714 -0.12857143 -0.11428571 -0.1 -0.08571429 -0.07142857 -0.05714286 -0.04285714 -0.02857143 -0.01428571 0 0 0 0 0 0
  line L19 (9.1664, -2.0687) -> (8.9139, -2.0117)
  arc A39 (8.6853, -1.6627) -> (8.9139, -2.0117) centre (8.9799, -1.7191) ccw
  arc A40 (8.6853, -1.6627) -> (8.774, -1.1026) centre (0, 0) ccw
  arc A41 (9.0993, -0.8413) -> (8.774, -1.1026) centre (9.0716, -1.14) ccw
  line L20 (9.0993, -0.8413) -> (9.357, -0.8651)
  spline S20 degree 5 poles (9.357, -0.8651) (9.3617, -0.8655) (9.371, -0.8663) (9.385, -0.867) (9.4037, -0.8673) (9.4271, -0.8667) (9.4506, -0.8654) (9.474, -0.8636) (9.4975, -0.8616) (9.5211, -0.8595) (9.5446, -0.8572) (9.5681, -0.8546) (9.5917, -0.8518) (9.6152, -0.8487) (9.6388, -0.8452) (9.6624, -0.8414) (9.686, -0.8373) (9.7095, -0.833) (9.7331, -0.8285) (9.7567, -0.8238) (9.7803, -0.8189) (9.8039, -0.8138) (9.8275, -0.8085) (9.8511, -0.803) (9.8747, -0.7973) (9.8983, -0.7914) (9.9219, -0.7853) (9.9454, -0.779) (9.969, -0.7725) (9.9926, -0.7658) (10.0162, -0.759) (10.0397, -0.752) (10.0633, -0.7448) (10.0868, -0.7375) (10.1104, -0.73) (10.1339, -0.7223) (10.1574, -0.7144) (10.181, -0.7064) (10.2045, -0.6982) (10.228, -0.6899) (10.2515, -0.6814) (10.2749, -0.6728) (10.2984, -0.664) (10.3218, -0.655) (10.3453, -0.6459) (10.3687, -0.6367) (10.3921, -0.6273) (10.4155, -0.6177) (10.4389, -0.608) (10.4623, -0.5982) (10.4857, -0.5882) (10.509, -0.578) (10.5323, -0.5678) (10.5556, -0.5573) (10.5789, -0.5468) (10.6022, -0.5361) (10.6255, -0.5252) (10.6487, -0.5143) (10.6719, -0.5032) (10.6951, -0.4919) (10.7183, -0.4805) (10.7415, -0.469) (10.7646, -0.4574) (10.7878, -0.4456) (10.8109, -0.4337) (10.834, -0.4216) (10.857, -0.4094) (10.8801, -0.3971) (10.9031, -0.3847) (10.9261, -0.3721) (10.9491, -0.3594) (10.9674, -0.3492) (10.9812, -0.3414) (10.9904, -0.3362) (10.9949, -0.3336) knots 0 0 0 0 0 0 0.01428571 0.02857143 0.04285714 0.05714286 0.07142857 0.08571429 0.1 0.11428571 0.12857143 0.14285714 0.15714286 0.17142857 0.18571429 0.2 0.21428571 0.22857143 0.24285714 0.25714286 0.27142857 0.28571429 0.3 0.31428571 0.32857143 0.34285714 0.35714286 0.37142857 0.38571429 0.4 0.41428571 0.42857143 0.44285714 0.45714286 0.47142857 0.48571429 0.5 0.51428571 0.52857143 0.54285714 0.55714286 0.57142857 0.58571429 0.6 0.61428571 0.62857143 0.64285714 0.65714286 0.67142857 0.68571429 0.7 0.71428571 0.72857143 0.74285714 0.75714286 0.77142857 0.78571429 0.8 0.81428571 0.82857143 0.84285714 0.85714286 0.87142857 0.88571429 0.9 0.91428571 0.92857143 0.94285714 0.95714286 0.97142857 0.98571429 1 1 1 1 1 1
  arc A42 (10.9949, -0.3336) -> (10.9949, 0.3336) centre (0, 0) ccw
  spline S21 degree 5 poles (10.9949, 0.3336) (10.9904, 0.3362) (10.9812, 0.3414) (10.9674, 0.3492) (10.9491, 0.3594) (10.9261, 0.3721) (10.9031, 0.3847) (10.8801, 0.3971) (10.857, 0.4094) (10.834, 0.4216) (10.8109, 0.4337) (10.7878, 0.4456) (10.7646, 0.4574) (10.7415, 0.469) (10.7183, 0.4805) (10.6951, 0.4919) (10.6719, 0.5032) (10.6487, 0.5143) (10.6255, 0.5252) (10.6022, 0.5361) (10.5789, 0.5468) (10.5556, 0.5573) (10.5323, 0.5678) (10.509, 0.578) (10.4857, 0.5882) (10.4623, 0.5982) (10.4389, 0.608) (10.4155, 0.6177) (10.3921, 0.6273) (10.3687, 0.6367) (10.3453, 0.6459) (10.3218, 0.655) (10.2984, 0.664) (10.2749, 0.6728) (10.2515, 0.6814) (10.228, 0.6899) (10.2045, 0.6982) (10.181, 0.7064) (10.1574, 0.7144) (10.1339, 0.7223) (10.1104, 0.73) (10.0868, 0.7375) (10.0633, 0.7448) (10.0397, 0.752) (10.0162, 0.759) (9.9926, 0.7658) (9.969, 0.7725) (9.9454, 0.779) (9.9219, 0.7853) (9.8983, 0.7914) (9.8747, 0.7973) (9.8511, 0.803) (9.8275, 0.8085) (9.8039, 0.8138) (9.7803, 0.8189) (9.7567, 0.8238) (9.7331, 0.8285) (9.7095, 0.833) (9.686, 0.8373) (9.6624, 0.8414) (9.6388, 0.8452) (9.6152, 0.8487) (9.5917, 0.8518) (9.5681, 0.8546) (9.5446, 0.8572) (9.5211, 0.8595) (9.4975, 0.8616) (9.474, 0.8636) (9.4506, 0.8654) (9.4271, 0.8667) (9.4037, 0.8673) (9.385, 0.867) (9.371, 0.8663) (9.3617, 0.8655) (9.357, 0.8651) knots -1 -1 -1 -1 -1 -1 -0.98571429 -0.97142857 -0.95714286 -0.94285714 -0.92857143 -0.91428571 -0.9 -0.88571429 -0.87142857 -0.85714286 -0.84285714 -0.82857143 -0.81428571 -0.8 -0.78571429 -0.77142857 -0.75714286 -0.74285714 -0.72857143 -0.71428571 -0.7 -0.68571429 -0.67142857 -0.65714286 -0.64285714 -0.62857143 -0.61428571 -0.6 -0.58571429 -0.57142857 -0.55714286 -0.54285714 -0.52857143 -0.51428571 -0.5 -0.48571429 -0.47142857 -0.45714286 -0.44285714 -0.42857143 -0.41428571 -0.4 -0.38571429 -0.37142857 -0.35714286 -0.34285714 -0.32857143 -0.31428571 -0.3 -0.28571429 -0.27142857 -0.25714286 -0.24285714 -0.22857143 -0.21428571 -0.2 -0.18571429 -0.17142857 -0.15714286 -0.14285714 -0.12857143 -0.11428571 -0.1 -0.08571429 -0.07142857 -0.05714286 -0.04285714 -0.02857143 -0.01428571 0 0 0 0 0 0
  line L21 (9.357, 0.8651) -> (9.0993, 0.8413)
  arc A43 (8.774, 1.1026) -> (9.0993, 0.8413) centre (9.0716, 1.14) ccw
  arc A44 (8.774, 1.1026) -> (8.6853, 1.6627) centre (0, 0) ccw
  arc A45 (8.9139, 2.0117) -> (8.6853, 1.6627) centre (8.9799, 1.7191) ccw
  line L22 (8.9139, 2.0117) -> (9.1664, 2.0687)
  spline S22 degree 5 poles (9.1664, 2.0687) (9.171, 2.0697) (9.1801, 2.0719) (9.1936, 2.0755) (9.2115, 2.0811) (9.2335, 2.0889) (9.2554, 2.0974) (9.2772, 2.1063) (9.299, 2.1154) (9.3207, 2.1248) (9.3423, 2.1342) (9.3639, 2.1439) (9.3855, 2.1539) (9.4069, 2.1641) (9.4282, 2.1747) (9.4495, 2.1856) (9.4706, 2.1968) (9.4917, 2.2082) (9.5128, 2.2198) (9.5338, 2.2315) (9.5547, 2.2435) (9.5755, 2.2556) (9.5964, 2.2679) (9.6171, 2.2805) (9.6378, 2.2932) (9.6584, 2.3061) (9.6789, 2.3192) (9.6994, 2.3325) (9.7198, 2.3459) (9.7402, 2.3595) (9.7605, 2.3733) (9.7807, 2.3873) (9.8009, 2.4014) (9.821, 2.4156) (9.8411, 2.43) (9.8611, 2.4446) (9.8811, 2.4594) (9.901, 2.4743) (9.9208, 2.4893) (9.9406, 2.5045) (9.9603, 2.5198) (9.9799, 2.5353) (9.9995, 2.5509) (10.0191, 2.5667) (10.0386, 2.5826) (10.058, 2.5986) (10.0773, 2.6148) (10.0966, 2.6311) (10.1159, 2.6476) (10.1351, 2.6642) (10.1542, 2.6809) (10.1733, 2.6977) (10.1923, 2.7147) (10.2112, 2.7318) (10.2301, 2.7491) (10.249, 2.7664) (10.2677, 2.7839) (10.2864, 2.8015) (10.3051, 2.8193) (10.3237, 2.8371) (10.3422, 2.8551) (10.3607, 2.8732) (10.3791, 2.8915) (10.3975, 2.9098) (10.4158, 2.9283) (10.434, 2.9469) (10.4522, 2.9656) (10.4703, 2.9844) (10.4883, 3.0034) (10.5063, 3.0224) (10.5242, 3.0416) (10.5385, 3.057) (10.5492, 3.0687) (10.5564, 3.0764) (10.5599, 3.0803) knots 0 0 0 0 0 0 0.01428571 0.02857143 0.04285714 0.05714286 0.07142857 0.08571429 0.1 0.11428571 0.12857143 0.14285714 0.15714286 0.17142857 0.18571429 0.2 0.21428571 0.22857143 0.24285714 0.25714286 0.27142857 0.28571429 0.3 0.31428571 0.32857143 0.34285714 0.35714286 0.37142857 0.38571429 0.4 0.41428571 0.42857143 0.44285714 0.45714286 0.47142857 0.48571429 0.5 0.51428571 0.52857143 0.54285714 0.55714286 0.57142857 0.58571429 0.6 0.61428571 0.62857143 0.64285714 0.65714286 0.67142857 0.68571429 0.7 0.71428571 0.72857143 0.74285714 0.75714286 0.77142857 0.78571429 0.8 0.81428571 0.82857143 0.84285714 0.85714286 0.87142857 0.88571429 0.9 0.91428571 0.92857143 0.94285714 0.95714286 0.97142857 0.98571429 1 1 1 1 1 1
  arc A46 (10.5599, 3.0803) -> (10.3537, 3.7149) centre (0, 0) ccw